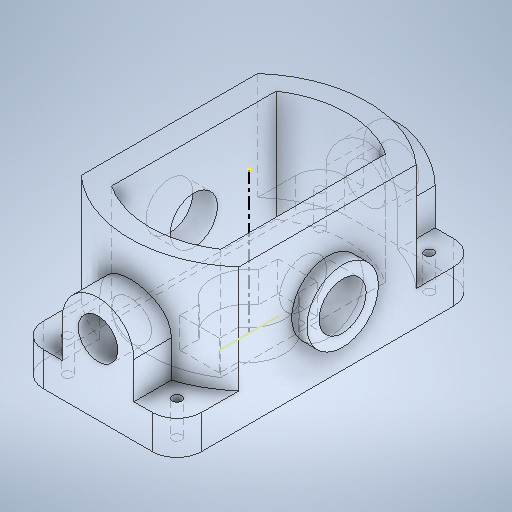
# Autodesk Inventor part: Bai_15
Saved by Autodesk Inventor 2025.1 (Build 291241000, 241)
## iProperties
Created: 2024-10-02
Part Number: Bai_15
Material: Generic
Document SubType Name: Modeling
Designer: msi
Density: 1 g/cm^3
Appearance: Default
Author: msi
Autodesk Inventor part; units mm, degrees
ref_plane "YZ Plane" through (0, 0, 0) normal (1, 0, 0) x (0, 1, 0)
ref_plane "XZ Plane" through (0, 0, 0) normal (0, 1, 0) x (-1, 0, 0)
ref_plane "XY Plane" through (0, 0, 0) normal (0, 0, 1) x (1, 0, 0)
sketch "Sketch1" plane through (0, 0, 0) normal (0, 1, 0) x (-1, 0, 0)
  circle A0 centre (0, 0) radius 19 construction
  line L0 (0, 0) -> (0, -26) construction
  line L1 (31.6894, 0) -> (-35.1324, 0) construction
  line L2 (0, 0) -> (0, 26) construction
  line L3 (0, -26) -> (10.5, -26)
  line L4 (0, -26) -> (-10.5, -26)
  line L5 (0, 26) -> (10.5, 26)
  line L6 (0, 26) -> (-10.5, 26)
  line L7 (10.5, 26) -> (10.5, -26) construction
  line L8 (-10.5, 26) -> (-10.5, -26) construction
  line L9 (10.5, 26) -> (10.5, 15.8351)
  line L10 (-10.5, 26) -> (-10.5, 15.8351)
  line L11 (10.5, -15.8351) -> (10.5, -26)
  line L12 (-10.5, -15.8351) -> (-10.5, -26)
  arc A1 (10.5, -15.8351) -> (10.5, 15.8351) centre (0, 0) ccw
  arc A2 (-10.5, 15.8351) -> (-10.5, -15.8351) centre (0, 0) ccw
  line L13 (-28.8775, 80) -> (29.1225, 80)
  line L14 (42.1225, 67) -> (42.1225, -67)
  line L15 (29.1225, -80) -> (-28.8775, -80)
  line L16 (-41.8775, -67) -> (-41.8775, 67)
  line L17 (66.9452, 0) -> (-66.7003, 0)
  line L18 (0.1225, 57.213) -> (0.1225, -133.7823)
  arc A3 (42.1225, 67) -> (29.1225, 80) centre (29.1225, 67) ccw
  arc A4 (29.1225, -80) -> (42.1225, -67) centre (29.1225, -67) ccw
  arc A5 (-41.8775, -67) -> (-28.8775, -80) centre (-28.8775, -67) ccw
  arc A6 (-28.8775, 80) -> (-41.8775, 67) centre (-28.8775, 67) ccw
  circle A7 centre (0, 0) radius 63 construction
  circle A8 centre (0, 0) radius 52.5 construction
  line L19 (-28.8775, -67) -> (29.1225, -67) construction
  line L20 (29.1225, -67) -> (29.1225, 67) construction
  line L21 (29.1225, 67) -> (-28.8775, 67) construction
  line L22 (-28.8775, 67) -> (-28.8775, -67) construction
  arc A9 (42.1225, 46.8476) -> (-41.8775, 47.0667) centre (0, 0) ccw
  arc A10 (-41.8775, -47.0667) -> (42.1225, -46.8476) centre (0, 0) ccw
  arc A11 (29.1225, 43.6822) -> (-28.8775, 43.8445) centre (0, 0) ccw
  arc A12 (-28.8775, -43.8445) -> (29.1225, -43.6822) centre (0, 0) ccw
  line L23 (29.1225, 43.6822) -> (29.1225, -43.6822)
  line L24 (-28.8775, 43.8445) -> (-28.8775, -43.8445)
  circle A13 centre (29.1225, -67) radius 2.5
  circle A14 centre (-28.8775, -67) radius 2.5
  circle A15 centre (29.1225, 67) radius 2.5
  circle A16 centre (-28.8775, 67) radius 2.5
  point P0 (-41.8775, 80)
  point P1 (42.1225, -80)
  point P2 (42.1225, 80)
  point P3 (-41.8775, -80)
  dimension "d0" = 38
  dimension "d3" = 10.5
  dimension "d4" = 10.5
  dimension "d5" = 84
  dimension "d6" = 160
  dimension "d7" = 13
  dimension "d10" = 126
  dimension "d11" = 105
  dimension "d12" = 58
  dimension "d13" = 134
  dimension "d20" = 5
  dimension "d21" = 5
  constraints: 50 end point, 33 point on circle, 20 point on line, 17 centre point, 11 coincident, 11 horizontal, 8 tangent, 6 symmetric about line, 6 vertical, 4 collinear, 4 parallel, 3 equal radius, 3 perpendicular, 2 other
  measures "d0" diameter of A0
  measures "d3" distance of L0.end L3.end
  measures "d4" distance of L0.end L4.end
  measures "d5" distance of point (42.122, -80) point (-41.878, -80)
  measures "d6" distance of point (-41.878, -80) point (-41.878, 80)
  measures "d7" radius of A3
  measures "d10" diameter of A7
  measures "d11" diameter of A8
  measures "d12" distance of L19.start L19.end
  measures "d13" distance of L19.end L20.end
  measures "d20" diameter of A13
  measures "d21" diameter of A14
extrude "Extrusion1" add sketch "Sketch1" against normal blind 75 contours L4 L12 A2 L17 L18 L3 | L3 L18 A12 L24 L17 A2 L12 L4 | L18 L17 A1 L11 L3 | L3 L11 A1 L17 L23 A12 L18 | L18 L5 L9 A1 L17 | L17 A2 L10 L6 L5 L18 | A12 L23 L17 L14 A10 L18 | L18 A10 L16 L17 L24 A12 | A1 L9 L5 L18 A11 L23 L17 | L17 L24 A11 L18 L5 L6 L10 A2 | A10 L14 A4 L15 L18 | L18 L15 A5 L16 A10 | L23 A11 L24 L17 L16 A9 L14 | A9 L16 A6 L13 A3 L14 | A13 | A14 | A15 | A16
extrude "Extrusion2" cut sketch "Sketch1" against normal blind 59 contours L3 L18 A12 L24 L17 A2 L12 L4 | L3 L11 A1 L17 L23 A12 L18 | A1 L9 L5 L18 A11 L23 L17 | L17 L24 A11 L18 L5 L6 L10 A2
extrude "Extrusion3" cut sketch "Sketch1" against normal blind 75 contours L4 L12 A2 L17 L18 L3 | L18 L17 A1 L11 L3 | L18 L5 L9 A1 L17 | L17 A2 L10 L6 L5 L18
extrude "Extrusion4" cut sketch "Sketch1" against normal blind 57 contours A10 L14 A4 L15 L18 | L18 L15 A5 L16 A10 | A9 L16 A6 L13 A3 L14 | A13 | A14 | A15 | A16
extrude "Extrusion5" cut sketch "Sketch1" against normal blind 75 contours A13 | A14 | A15 | A16
sketch "Sketch2" plane through (0, 0, 0) normal (1, 0, 0) x (0, 1, 0)
  line L0 (0, 0) -> (-75, 0)
  line L1 (-75, -15.8351) -> (-75, 15.8351) projected
  constraints: 2 end point, 1 midpoint
sketch "Sketch3" plane through (41.8775, -75, 67) normal (1, 0, 0) x (0, 0, -1)
  line L0 (67, 75) -> (67, 0)
  line L1 (82.8351, 0) -> (51.1649, 0) projected
  circle A0 centre (67, 37.5) radius 12.5
  circle A1 centre (67, 37.5) radius 19
  dimension "d24" = 25
  dimension "d25" = 38
  constraints: 2 centre point, 2 end point, 2 midpoint, 1 coincident
  measures "d24" diameter of A0
  measures "d25" diameter of A1
extrude "Extrusion6" cut sketch "Sketch3" against normal blind 84 contours A0 L0 | L0 A0
sketch "Sketch4" plane through (0, 0, 0) normal (1, 0, 0) x (0, 1, 0)
  point P0 (0, 0)
sketch "Sketch5" plane through (0, 0, 0) normal (1, 0, 0) x (0, 1, 0)
  point P0 (0, 0)
sketch "Sketch6" plane through (41.8775, -75, 67) normal (1, 0, 0) x (0, 0, -1)
  circle A0 centre (67, 37.5) radius 12.5 projected
  circle A1 centre (67, 37.5) radius 19
  point P0 (67, 75)
  dimension "d28" = 38
  constraints: 1 centre point, 1 coincident
  measures "d28" diameter of A1
extrude "Extrusion7" add sketch "Sketch6" along normal blind 8
sketch "Sketch7" plane through (28.8775, -75, -80) normal (0, 0, -1) x (-1, 0, 0)
  line L0 (28.8775, 75) -> (28.8775, 0)
  circle A0 centre (28.8775, 37.5) radius 10.5
  circle A1 centre (28.8775, 37.5) radius 19 construction
  line L1 (9.8775, 37.5) -> (9.8775, 18)
  line L2 (0, 18) -> (58, 18) projected
  line L3 (47.8775, 37.5) -> (47.8775, 18)
  arc A2 (47.8775, 37.5) -> (9.8775, 37.5) centre (28.8775, 37.5) ccw
  dimension "d31" = 21
  dimension "d32" = 38
  constraints: 6 end point, 4 point on circle, 3 centre point, 3 vertical, 2 coincident, 2 point on line, 1 midpoint, 1 parallel, 1 tangent, 1 other
  measures "d31" diameter of A0
  measures "d32" diameter of A1
extrude "Extrusion8" add sketch "Sketch7" against normal blind 160 contours A2 L3 L2 L0 A0 | L0 A0 L2 L1 A2
extrude "Extrusion9" cut sketch "Sketch1" against normal blind 75 contours L4 L12 A2 L17 L18 L3 | L18 L17 A1 L11 L3 | L18 L5 L9 A1 L17 | L17 A2 L10 L6 L5 L18
extrude "Extrusion10" cut sketch "Sketch1" against normal blind 59 contours L3 L18 A12 L24 L17 A2 L12 L4 | L3 L11 A1 L17 L23 A12 L18 | A1 L9 L5 L18 A11 L23 L17 | L17 L24 A11 L18 L5 L6 L10 A2
body "Solid1"
